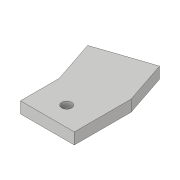
# Autodesk Inventor part: Lidar Sensor CAse Piece 1
Saved by Autodesk Inventor 2018.3 (Build 223284000, 284)
## iProperties
Created: 2019-02-15
Part Number: Lidar Sensor CAse Piece 1
Material: Generic
Document SubType Name: Modeling
Designer: aye06091
Mass: 6.62267 g
Surface Area: 34.7847 cm^2
Volume: 6.62267 cm^3
Density: 1 g/cm^3
Appearance: Default
Author: aye06091
Autodesk Inventor part; units mm, degrees
ref_plane "YZ Plane" through (0, 0, 0) normal (1, 0, 0) x (0, 1, 0)
ref_plane "XZ Plane" through (0, 0, 0) normal (0, 1, 0) x (-1, 0, 0)
ref_plane "XY Plane" through (0, 0, 0) normal (0, 0, 1) x (1, 0, 0)
sketch "Sketch1" plane through (0, 0, 0) normal (0, 1, 0) x (-1, 0, 0)
  line L0 (-8.0312, -19.6194) -> (-8.0312, -0.5694)
  line L1 (-8.0312, -0.5694) -> (-34.5277, -0.5694)
  line L2 (-34.5277, -0.5694) -> (-34.5277, -28.5056)
  line L3 (18.6455, 5.0782) -> (18.6456, 5.0782)
  line L4 (-1.974, -37.6808) -> (-8.0312, -19.6194)
  line L5 (-34.5277, -28.5056) -> (-27.4611, -49.5771)
  line L6 (-1.974, -37.6808) -> (-0.9645, -40.691)
  line L7 (-27.4611, -49.5771) -> (-0.9645, -40.691)
  circle A0 centre (-21.2794, -10.0945) radius 2.4447
  line L8 (-8.0312, -0.5694) -> (-8.0312, -19.6194)
  line L9 (-8.0312, -19.6194) -> (-0.9645, -40.691)
  line L10 (-0.9645, -40.691) -> (-27.4611, -49.5771)
  line L11 (-27.4611, -49.5771) -> (-34.5277, -28.5056)
  line L12 (-34.5277, -28.5056) -> (-34.5277, -0.5694)
  line L13 (-34.5277, -0.5694) -> (-8.0312, -0.5694)
  dimension "d0" = 19.05
  dimension "d1" = 22.225
  dimension "d2" = 27.9469
  dimension "d3" = 26.4965
  dimension "d4" = 4.8895
  dimension "d18" = 13.2483
  dimension "d19" = 9.525
  dimension "d20" = 161.46
  constraints: 28 end point, 3 perpendicular, 2 parallel, 1 centre point, 1 collinear, 1 vertical
  measures "d0" distance of L0.start L0.end
  measures "d1" distance of L4.end L6.end
  measures "d2" distance of L5.end L7.end
  measures "d3" distance of L0.end L1.end
  measures "d4" diameter of A0
  measures "d18" distance from line of A0.centre L2
  measures "d19" distance from line of A0.centre L1
  measures "d20" angle of L4 L0
extrude "Extrusion1" add sketch "Sketch1" along normal blind 5.588
sketch "Sketch2" plane through (0, 0, 0) normal (0, -1, 0) x (1, 0, 0)
  line L0 (27.4611, -49.5771) -> (0.9645, -40.691) projected
  line L1 (31.5175, -27.4959) -> (29.9883, -26.9832)
  line L2 (34.5277, -28.5056) -> (27.4611, -49.5771) projected
  line L3 (27.4611, -49.5771) -> (0.9645, -40.691) projected
  line L4 (31.5175, -27.4959) -> (8.0312, -19.6194)
  line L5 (8.0312, -19.6194) -> (7.0136, -22.6537)
  line L6 (7.0136, -22.6537) -> (27.4656, -29.5126)
  line L7 (24.4508, -48.5675) -> (21.4165, -47.5499)
  line L8 (21.4165, -47.5499) -> (27.4656, -29.5126)
  line L9 (29.9883, -26.9831) -> (31.5175, -27.4959)
  line L10 (31.5175, -27.4959) -> (24.4508, -48.5675)
  point P0 (0, 0)
  dimension "d15" = 3.2004
  dimension "d16" = 3.175
  dimension "d17" = 3.2004
  constraints: 16 end point, 3 parallel, 3 perpendicular, 2 point on line
  measures "d15" distance between parallel lines of L4 L6
  measures "d16" distance between parallel lines of L2 L10
  measures "d17" distance between parallel lines of L8 L10
extrude "Extrusion2" cut sketch "Sketch2" against normal blind 1.5875
fillet "Fillet1" radius 1.5875 1 edges at (31.5175, 0.7937, -27.4959)
body "Solid1"
